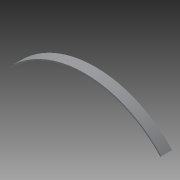
# Autodesk Inventor part: Shooter_4inRollerGuide20160126
Saved by Autodesk Inventor 2014 (Build 180170000, 170)
## iProperties
Created: 2016-01-26
Part Number: Shooter_4inRollerGuide20160126
Material: Generic
Document SubType Name: Modeling
Designer: choices
Density: 1 g/cm^3
Appearance: Default
Author: choices
Autodesk Inventor part; units mm, degrees
ref_plane "YZ Plane" through (0, 0, 0) normal (1, 0, 0) x (0, 1, 0)
ref_plane "XZ Plane" through (0, 0, 0) normal (0, 1, 0) x (-1, 0, 0)
ref_plane "XY Plane" through (0, 0, 0) normal (0, 0, 1) x (1, 0, 0)
sketch "Sketch1" plane through (0, 0, 0) normal (0, 0, 1) x (1, 0, 0)
  line L0 (0, 0) -> (355.6, 0)
  arc A0 (355.6, 0) -> (0, 0) centre (177.8, -163.1345) ccw
  circle A1 centre (177.8, -163.1345) radius 244.475
  line L1 (177.8, -163.1345) -> (355.6, 0)
  line L2 (177.8, -163.1345) -> (0, 0)
  line L3 (0, 0) -> (-2.3395, 2.1465)
  line L4 (355.6, 0) -> (357.9395, 2.1465)
  dimension "d0" = 355.6
  dimension "d1" = 241.3
  dimension "d5" = 488.95
  constraints: 10 end point, 4 point on circle, 2 centre point, 2 collinear, 1 coincident, 1 horizontal
  measures "d0" distance of L0.start L0.end
  measures "d1" radius of A0
  measures "d5" diameter of A1
extrude "Extrusion1" add sketch "Sketch1" along normal blind 25.4 contours L3 A1 L4 A0
body "Solid1"
